Autodesk Fusion 360 part; units mm, degrees
note: some values were not read from the file. Chosen so that the rebuilt part matches the saved one: which face or edge a step refers to; a direction.
(part 2 of 2)
sketch "Esquisse21" plane through (120, 0, 0) normal (1, 0, 0) x (0, 0, -1)
  line L0 (3, 100) -> (3, 3)
  line L1 (3, 3) -> (167, 3)
  line L2 (167, 3) -> (167, 100)
  line L3 (167, 100) -> (3, 100)
  line L4 (3, 100) -> (85, 100)
  line L5 (85, 52) -> (87.5981, 53.5)
  line L6 (87.5981, 53.5) -> (87.5981, 56.5)
  line L7 (87.5981, 56.5) -> (85, 58)
  line L8 (85, 58) -> (82.4019, 56.5)
  line L9 (82.4019, 56.5) -> (82.4019, 53.5)
  line L10 (82.4019, 53.5) -> (85, 52)
  line L11 (68.0981, 56.5) -> (65.5, 58)
  line L12 (65.5, 58) -> (62.9019, 56.5)
  line L13 (62.9019, 56.5) -> (62.9019, 53.5)
  line L14 (62.9019, 53.5) -> (65.5, 52)
  line L15 (65.5, 52) -> (68.0981, 53.5)
  line L16 (68.0981, 53.5) -> (68.0981, 56.5)
  line L17 (74.5981, 56.5) -> (72, 58)
  line L18 (72, 58) -> (69.4019, 56.5)
  line L19 (69.4019, 56.5) -> (69.4019, 53.5)
  line L20 (69.4019, 53.5) -> (72, 52)
  line L21 (72, 52) -> (74.5981, 53.5)
  line L22 (74.5981, 53.5) -> (74.5981, 56.5)
  line L23 (81.0981, 56.5) -> (78.5, 58)
  line L24 (78.5, 58) -> (75.9019, 56.5)
  line L25 (75.9019, 56.5) -> (75.9019, 53.5)
  line L26 (75.9019, 53.5) -> (78.5, 52)
  line L27 (78.5, 52) -> (81.0981, 53.5)
  line L28 (81.0981, 53.5) -> (81.0981, 56.5)
  line L29 (94.0981, 56.5) -> (91.5, 58)
  line L30 (91.5, 58) -> (88.9019, 56.5)
  line L31 (88.9019, 56.5) -> (88.9019, 53.5)
  line L32 (88.9019, 53.5) -> (91.5, 52)
  line L33 (91.5, 52) -> (94.0981, 53.5)
  line L34 (94.0981, 53.5) -> (94.0981, 56.5)
  line L35 (100.5981, 56.5) -> (98, 58)
  line L36 (98, 58) -> (95.4019, 56.5)
  line L37 (95.4019, 56.5) -> (95.4019, 53.5)
  line L38 (95.4019, 53.5) -> (98, 52)
  line L39 (98, 52) -> (100.5981, 53.5)
  line L40 (100.5981, 53.5) -> (100.5981, 56.5)
  line L41 (107.0981, 56.5) -> (104.5, 58)
  line L42 (104.5, 58) -> (101.9019, 56.5)
  line L43 (101.9019, 56.5) -> (101.9019, 53.5)
  line L44 (101.9019, 53.5) -> (104.5, 52)
  line L45 (104.5, 52) -> (107.0981, 53.5)
  line L46 (107.0981, 53.5) -> (107.0981, 56.5)
  line L47 (113.5981, 56.5) -> (111, 58)
  line L48 (111, 58) -> (108.4019, 56.5)
  line L49 (108.4019, 56.5) -> (108.4019, 53.5)
  line L50 (108.4019, 53.5) -> (111, 52)
  line L51 (111, 52) -> (113.5981, 53.5)
  line L52 (113.5981, 53.5) -> (113.5981, 56.5)
  line L53 (68.0981, 50) -> (65.5, 51.5)
  line L54 (65.5, 51.5) -> (62.9019, 50)
  line L55 (62.9019, 50) -> (62.9019, 47)
  line L56 (62.9019, 47) -> (65.5, 45.5)
  line L57 (65.5, 45.5) -> (68.0981, 47)
  line L58 (68.0981, 47) -> (68.0981, 50)
  line L59 (74.5981, 50) -> (72, 51.5)
  line L60 (72, 51.5) -> (69.4019, 50)
  line L61 (69.4019, 50) -> (69.4019, 47)
  line L62 (69.4019, 47) -> (72, 45.5)
  line L63 (72, 45.5) -> (74.5981, 47)
  line L64 (74.5981, 47) -> (74.5981, 50)
  line L65 (81.0981, 50) -> (78.5, 51.5)
  line L66 (78.5, 51.5) -> (75.9019, 50)
  line L67 (75.9019, 50) -> (75.9019, 47)
  line L68 (75.9019, 47) -> (78.5, 45.5)
  line L69 (78.5, 45.5) -> (81.0981, 47)
  line L70 (81.0981, 47) -> (81.0981, 50)
  line L71 (87.5981, 50) -> (85, 51.5)
  line L72 (85, 51.5) -> (82.4019, 50)
  line L73 (82.4019, 50) -> (82.4019, 47)
  line L74 (82.4019, 47) -> (85, 45.5)
  line L75 (85, 45.5) -> (87.5981, 47)
  line L76 (87.5981, 47) -> (87.5981, 50)
  line L77 (94.0981, 50) -> (91.5, 51.5)
  line L78 (91.5, 51.5) -> (88.9019, 50)
  line L79 (88.9019, 50) -> (88.9019, 47)
  line L80 (88.9019, 47) -> (91.5, 45.5)
  line L81 (91.5, 45.5) -> (94.0981, 47)
  line L82 (94.0981, 47) -> (94.0981, 50)
  line L83 (100.5981, 50) -> (98, 51.5)
  line L84 (98, 51.5) -> (95.4019, 50)
  line L85 (95.4019, 50) -> (95.4019, 47)
  line L86 (95.4019, 47) -> (98, 45.5)
  line L87 (98, 45.5) -> (100.5981, 47)
  line L88 (100.5981, 47) -> (100.5981, 50)
  line L89 (107.0981, 50) -> (104.5, 51.5)
  line L90 (104.5, 51.5) -> (101.9019, 50)
  line L91 (101.9019, 50) -> (101.9019, 47)
  line L92 (101.9019, 47) -> (104.5, 45.5)
  line L93 (104.5, 45.5) -> (107.0981, 47)
  line L94 (107.0981, 47) -> (107.0981, 50)
  line L95 (113.5981, 50) -> (111, 51.5)
  line L96 (111, 51.5) -> (108.4019, 50)
  line L97 (108.4019, 50) -> (108.4019, 47)
  line L98 (108.4019, 47) -> (111, 45.5)
  line L99 (111, 45.5) -> (113.5981, 47)
  line L100 (113.5981, 47) -> (113.5981, 50)
  line L101 (68.0981, 43.5) -> (65.5, 45)
  line L102 (65.5, 45) -> (62.9019, 43.5)
  line L103 (62.9019, 43.5) -> (62.9019, 40.5)
  line L104 (62.9019, 40.5) -> (65.5, 39)
  line L105 (65.5, 39) -> (68.0981, 40.5)
  line L106 (68.0981, 40.5) -> (68.0981, 43.5)
  line L107 (74.5981, 43.5) -> (72, 45)
  line L108 (72, 45) -> (69.4019, 43.5)
  line L109 (69.4019, 43.5) -> (69.4019, 40.5)
  line L110 (69.4019, 40.5) -> (72, 39)
  line L111 (72, 39) -> (74.5981, 40.5)
  line L112 (74.5981, 40.5) -> (74.5981, 43.5)
  line L113 (81.0981, 43.5) -> (78.5, 45)
  line L114 (78.5, 45) -> (75.9019, 43.5)
  line L115 (75.9019, 43.5) -> (75.9019, 40.5)
  line L116 (75.9019, 40.5) -> (78.5, 39)
  line L117 (78.5, 39) -> (81.0981, 40.5)
  line L118 (81.0981, 40.5) -> (81.0981, 43.5)
  line L119 (87.5981, 43.5) -> (85, 45)
  line L120 (85, 45) -> (82.4019, 43.5)
  line L121 (82.4019, 43.5) -> (82.4019, 40.5)
  line L122 (82.4019, 40.5) -> (85, 39)
  line L123 (85, 39) -> (87.5981, 40.5)
  line L124 (87.5981, 40.5) -> (87.5981, 43.5)
  line L125 (94.0981, 43.5) -> (91.5, 45)
  line L126 (91.5, 45) -> (88.9019, 43.5)
  line L127 (88.9019, 43.5) -> (88.9019, 40.5)
  line L128 (88.9019, 40.5) -> (91.5, 39)
  line L129 (91.5, 39) -> (94.0981, 40.5)
  line L130 (94.0981, 40.5) -> (94.0981, 43.5)
  line L131 (100.5981, 43.5) -> (98, 45)
  line L132 (98, 45) -> (95.4019, 43.5)
  line L133 (95.4019, 43.5) -> (95.4019, 40.5)
  line L134 (95.4019, 40.5) -> (98, 39)
  line L135 (98, 39) -> (100.5981, 40.5)
  line L136 (100.5981, 40.5) -> (100.5981, 43.5)
  line L137 (107.0981, 43.5) -> (104.5, 45)
  line L138 (104.5, 45) -> (101.9019, 43.5)
  line L139 (101.9019, 43.5) -> (101.9019, 40.5)
  line L140 (101.9019, 40.5) -> (104.5, 39)
  line L141 (104.5, 39) -> (107.0981, 40.5)
  line L142 (107.0981, 40.5) -> (107.0981, 43.5)
  line L143 (113.5981, 43.5) -> (111, 45)
  line L144 (111, 45) -> (108.4019, 43.5)
  line L145 (108.4019, 43.5) -> (108.4019, 40.5)
  line L146 (108.4019, 40.5) -> (111, 39)
  line L147 (111, 39) -> (113.5981, 40.5)
  line L148 (113.5981, 40.5) -> (113.5981, 43.5)
  line L149 (68.0981, 37) -> (65.5, 38.5)
  line L150 (65.5, 38.5) -> (62.9019, 37)
  line L151 (62.9019, 37) -> (62.9019, 34)
  line L152 (62.9019, 34) -> (65.5, 32.5)
  line L153 (65.5, 32.5) -> (68.0981, 34)
  line L154 (68.0981, 34) -> (68.0981, 37)
  line L155 (74.5981, 37) -> (72, 38.5)
  line L156 (72, 38.5) -> (69.4019, 37)
  line L157 (69.4019, 37) -> (69.4019, 34)
  line L158 (69.4019, 34) -> (72, 32.5)
  line L159 (72, 32.5) -> (74.5981, 34)
  line L160 (74.5981, 34) -> (74.5981, 37)
  line L161 (81.0981, 37) -> (78.5, 38.5)
  line L162 (78.5, 38.5) -> (75.9019, 37)
  line L163 (75.9019, 37) -> (75.9019, 34)
  line L164 (75.9019, 34) -> (78.5, 32.5)
  line L165 (78.5, 32.5) -> (81.0981, 34)
  line L166 (81.0981, 34) -> (81.0981, 37)
  line L167 (87.5981, 37) -> (85, 38.5)
  line L168 (85, 38.5) -> (82.4019, 37)
  line L169 (82.4019, 37) -> (82.4019, 34)
  line L170 (82.4019, 34) -> (85, 32.5)
  line L171 (85, 32.5) -> (87.5981, 34)
  line L172 (87.5981, 34) -> (87.5981, 37)
  line L173 (94.0981, 37) -> (91.5, 38.5)
  line L174 (91.5, 38.5) -> (88.9019, 37)
  line L175 (88.9019, 37) -> (88.9019, 34)
  line L176 (88.9019, 34) -> (91.5, 32.5)
  line L177 (91.5, 32.5) -> (94.0981, 34)
  line L178 (94.0981, 34) -> (94.0981, 37)
  line L179 (100.5981, 37) -> (98, 38.5)
  line L180 (98, 38.5) -> (95.4019, 37)
  line L181 (95.4019, 37) -> (95.4019, 34)
  line L182 (95.4019, 34) -> (98, 32.5)
  line L183 (98, 32.5) -> (100.5981, 34)
  line L184 (100.5981, 34) -> (100.5981, 37)
  line L185 (107.0981, 37) -> (104.5, 38.5)
  line L186 (104.5, 38.5) -> (101.9019, 37)
  line L187 (101.9019, 37) -> (101.9019, 34)
  line L188 (101.9019, 34) -> (104.5, 32.5)
  line L189 (104.5, 32.5) -> (107.0981, 34)
  line L190 (107.0981, 34) -> (107.0981, 37)
  line L191 (113.5981, 37) -> (111, 38.5)
  line L192 (111, 38.5) -> (108.4019, 37)
  line L193 (108.4019, 37) -> (108.4019, 34)
  line L194 (108.4019, 34) -> (111, 32.5)
  line L195 (111, 32.5) -> (113.5981, 34)
  line L196 (113.5981, 34) -> (113.5981, 37)
  line L197 (68.0981, 30.5) -> (65.5, 32)
  line L198 (65.5, 32) -> (62.9019, 30.5)
  line L199 (62.9019, 30.5) -> (62.9019, 27.5)
  line L200 (62.9019, 27.5) -> (65.5, 26)
  line L201 (65.5, 26) -> (68.0981, 27.5)
  line L202 (68.0981, 27.5) -> (68.0981, 30.5)
  line L203 (74.5981, 30.5) -> (72, 32)
  line L204 (72, 32) -> (69.4019, 30.5)
  line L205 (69.4019, 30.5) -> (69.4019, 27.5)
  line L206 (69.4019, 27.5) -> (72, 26)
  line L207 (72, 26) -> (74.5981, 27.5)
  line L208 (74.5981, 27.5) -> (74.5981, 30.5)
  line L209 (81.0981, 30.5) -> (78.5, 32)
  line L210 (78.5, 32) -> (75.9019, 30.5)
  line L211 (75.9019, 30.5) -> (75.9019, 27.5)
  line L212 (75.9019, 27.5) -> (78.5, 26)
  line L213 (78.5, 26) -> (81.0981, 27.5)
  line L214 (81.0981, 27.5) -> (81.0981, 30.5)
  line L215 (87.5981, 30.5) -> (85, 32)
  line L216 (85, 32) -> (82.4019, 30.5)
  line L217 (82.4019, 30.5) -> (82.4019, 27.5)
  line L218 (82.4019, 27.5) -> (85, 26)
  line L219 (85, 26) -> (87.5981, 27.5)
  line L220 (87.5981, 27.5) -> (87.5981, 30.5)
  line L221 (94.0981, 30.5) -> (91.5, 32)
  line L222 (91.5, 32) -> (88.9019, 30.5)
  line L223 (88.9019, 30.5) -> (88.9019, 27.5)
  line L224 (88.9019, 27.5) -> (91.5, 26)
  line L225 (91.5, 26) -> (94.0981, 27.5)
  line L226 (94.0981, 27.5) -> (94.0981, 30.5)
  line L227 (100.5981, 30.5) -> (98, 32)
  line L228 (98, 32) -> (95.4019, 30.5)
  line L229 (95.4019, 30.5) -> (95.4019, 27.5)
  line L230 (95.4019, 27.5) -> (98, 26)
  line L231 (98, 26) -> (100.5981, 27.5)
  line L232 (100.5981, 27.5) -> (100.5981, 30.5)
  line L233 (107.0981, 30.5) -> (104.5, 32)
  line L234 (104.5, 32) -> (101.9019, 30.5)
  line L235 (101.9019, 30.5) -> (101.9019, 27.5)
  line L236 (101.9019, 27.5) -> (104.5, 26)
  line L237 (104.5, 26) -> (107.0981, 27.5)
  line L238 (107.0981, 27.5) -> (107.0981, 30.5)
  line L239 (113.5981, 30.5) -> (111, 32)
  line L240 (111, 32) -> (108.4019, 30.5)
  line L241 (108.4019, 30.5) -> (108.4019, 27.5)
  line L242 (108.4019, 27.5) -> (111, 26)
  line L243 (111, 26) -> (113.5981, 27.5)
  line L244 (113.5981, 27.5) -> (113.5981, 30.5)
  point P0 (85, 55)
  dimension "d165" = 26
  dimension "d166" = -26
  constraint coincident L0.start L3.end
  constraint midpoint L3 L4.end
move_body "Déplacer1" bodies 1 to x (1, 0, 0) y (0, 1, 0) z (0, 0, 1) at (170, 150, 0)
move_body "Déplacer2" bodies 1 to x (1, 0, 0) y (0, 1, 0) z (0, 0, 1) at (-150, -50, 0)
extrude "Extrusion35" cut 2 faces at (-91.8333, 103.3333, -133) (-91.8333, 103.3333, -133) along direction (0, 0, 1) blind 15
fillet "Congé5" radius 3 8 edges at (-30, 101, -170) (-30.8787, 104.1213, -169.1213) (-150, 101, -170) (-149.1213, 104.1213, -169.1213) (-150, 101, 0) (-149.1213, 104.1213, -0.8787) (-30, 101, 0) (-30.8787, 104.1213, -0.8787)
equation "d26 = 'OUTPUT'"
equation "d36 = 'INPUT'"
